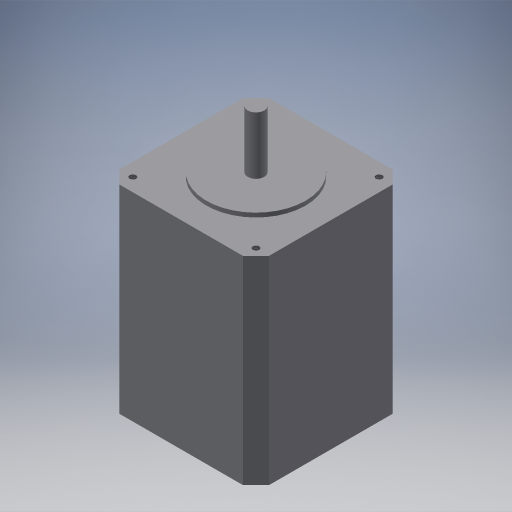
# Autodesk Inventor part: Motor ST nema 23
Saved by Autodesk Inventor 2024.3 (Build 283343000, 343)
## iProperties
Created: 2024-05-29
Part Number: Motor ST nema 23
Material: Allgemein
Document SubType Name: Modeling
Designer: Vogel
Density: 1 g/cm^3
Appearance: Vorgabe
Author: Vogel
Autodesk Inventor part; units mm, degrees
ref_plane "YZ Plane" through (0, 0, 0) normal (1, 0, 0) x (0, 1, 0)
ref_plane "XZ Plane" through (0, 0, 0) normal (0, 1, 0) x (-1, 0, 0)
ref_plane "XY Plane" through (0, 0, 0) normal (0, 0, 1) x (1, 0, 0)
sketch "Skizze1" plane through (0, 0, 0) normal (0, 0, 1) x (1, 0, 0)
  line L0 (-40.11, 0) -> (40.11, 0) projected
  line L1 (0, -40.11) -> (0, 40.11) projected
  line L2 (28.65, -28.65) -> (-28.65, -28.65)
  line L3 (-28.65, -28.65) -> (-28.65, 28.65)
  line L4 (-28.65, 28.65) -> (28.65, 28.65)
  line L5 (28.65, 28.65) -> (28.65, -28.65)
  line L6 (28.65, -28.65) -> (-28.65, 28.65) construction
  line L7 (-28.65, -28.65) -> (28.65, 28.65) construction
  point P0 (0, 0)
  dimension "d0" = 57.3
  dimension "d1" = 57.3
  constraints: 12 end point, 2 midpoint, 2 parallel, 1 horizontal, 1 perpendicular
  measures "d0" distance of L3.end L4.end
  measures "d1" distance of L2.end L3.end
extrude "Extrusion1" add sketch "Skizze1" along normal blind 76
sketch "Skizze2" plane through (0, 0, 76) normal (0, 0, 1) x (1, 0, 0)
  circle A0 centre (0, 0) radius 19
  dimension "d4" = 38
  constraints: 1 centre point, 1 coincident
  measures "d4" diameter of A0
extrude "Extrusion2" add sketch "Skizze2" along normal blind 1.6
sketch "Skizze3" plane through (0, 0, 77.6) normal (0, 0, 1) x (1, 0, 0)
  circle A0 centre (0, 0) radius 3.175
  dimension "d7" = 6.35
  constraints: 1 centre point, 1 coincident
  measures "d7" diameter of A0
extrude "Extrusion3" add sketch "Skizze3" along normal blind 22
sketch "Skizze4" plane through (0, 0, 76) normal (0, 0, 1) x (1, 0, 0)
  circle A0 centre (0, 0) radius 19 projected
  line L0 (28.65, 28.65) -> (-28.65, 28.65) projected
  line L1 (-28.65, 28.65) -> (-28.65, -28.65) projected
  line L2 (-28.65, -28.65) -> (28.65, -28.65) projected
  line L3 (28.65, -28.65) -> (28.65, 28.65) projected
  line L4 (23.575, -23.575) -> (-23.575, -23.575)
  line L5 (-23.575, -23.575) -> (-23.575, 23.575)
  line L6 (-23.575, 23.575) -> (23.575, 23.575)
  line L7 (23.575, 23.575) -> (23.575, -23.575)
  line L8 (23.575, -23.575) -> (-23.575, 23.575) construction
  line L9 (-23.575, -23.575) -> (23.575, 23.575) construction
  dimension "d10" = 47.15
  dimension "d11" = 47.15
  constraints: 12 end point, 4 coincident, 2 midpoint, 2 parallel, 1 horizontal, 1 perpendicular
  measures "d10" distance of L5.end L6.end
  measures "d11" distance of L4.end L5.end
hole "Bohrung1" at (-23.575, 23.575, 76) at (23.575, 23.575, 76) at (23.575, -23.575, 76) at (-23.575, -23.575, 76) direction (0, 0, -1) diameter 2.459 depth 8.8 tip angle 118 thread size "M3x0.5" class "6H" standard "ISO Metric profile"
chamfer "Fasen1" distance 5 angle 45 4 edges at (28.65, -28.65, 38) (28.65, 28.65, 38) (-28.65, 28.65, 38) (-28.65, -28.65, 38)
equation "\"d1\" = d0"
equation "\"d11\" = d10"
